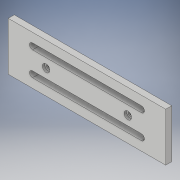
# Autodesk Inventor part: ps bottom
Saved by Autodesk Inventor 2017 (Build 210142000, 142)
## iProperties
Created: 2016-07-21
Part Number: ps bottom
Material: Generic
Document SubType Name: Modeling
Designer: Darien Morrow
Density: 1 g/cm^3
Appearance: Default
Author: Darien Morrow
Autodesk Inventor part; units mm, degrees
ref_plane "YZ Plane" through (0, 0, 0) normal (1, 0, 0) x (0, 1, 0)
ref_plane "XZ Plane" through (0, 0, 0) normal (0, 1, 0) x (-1, 0, 0)
ref_plane "XY Plane" through (0, 0, 0) normal (0, 0, 1) x (1, 0, 0)
sketch "Sketch1" plane through (0, 0, 0) normal (0, 0, 1) x (1, 0, 0)
  line L0 (0, 0) -> (165.1, 0)
  line L1 (165.1, 0) -> (165.1, 50.8)
  line L2 (165.1, 50.8) -> (0, 50.8)
  line L3 (0, 50.8) -> (0, 0)
  dimension "d0" = 165.1
  dimension "d1" = 50.8
  constraints: 8 end point, 2 parallel, 1 horizontal, 1 perpendicular
  measures "d0" distance between parallel lines of L1 L3
  measures "d1" distance between parallel lines of L0 L2
extrude "Extrusion1" add sketch "Sketch1" along normal blind 6.35
sketch "Sketch3" plane through (0, 0, 6.35) normal (0, 0, 1) x (1, 0, 0)
  line L0 (39.6875, 25.4) -> (125.4125, 25.4)
  line L1 (0, 0) -> (165.1, 0) projected
  line L2 (0, 50.8) -> (0, 0) projected
  line L3 (165.1, 50.8) -> (0, 50.8) projected
  line L4 (82.55, 50.8) -> (82.55, 0)
  line L5 (165.1, 0) -> (165.1, 50.8) projected
  dimension "d14" = 85.725
  dimension "d15" = 25.4
  dimension "d16" = 39.6875
  dimension "d33" = 165.1
  dimension "d34" = 39.6875
  constraints: 4 end point, 2 coincident, 2 midpoint, 1 horizontal
  measures "d14" distance of L0.end L0.start
  measures "d15" distance between parallel lines of L0 L1
  measures "d16" distance from line of L0.start L2
  measures "d33" distance of L1.start L1.end
  measures "d34" distance from line of L5 L0.end
hole "Hole1" at (39.6875, 25.4, 6.35) at (125.4125, 25.4, 6.35) direction (0, 0, -1) diameter 4.1656 depth 6.35 tip angle 118 counterbore diameter 7.9502 counterbore depth 2.54
sketch "Sketch4" plane through (0, 0, 0) normal (0, 0, -1) x (-1, 0, 0)
  line L0 (-139.7, 12.7) -> (-25.4, 12.7) construction
  line L1 (-139.7, 9.525) -> (-25.4, 9.525)
  line L2 (-25.4, 15.875) -> (-139.7, 15.875)
  arc A0 (-139.7, 15.875) -> (-139.7, 9.525) centre (-139.7, 12.7) ccw
  arc A1 (-25.4, 9.525) -> (-25.4, 15.875) centre (-25.4, 12.7) ccw
  line L3 (0, 50.8) -> (0, 0) projected
  line L4 (-139.7, 38.1) -> (-25.4, 38.1) construction
  line L5 (-139.7, 34.925) -> (-25.4, 34.925)
  line L6 (-25.4, 41.275) -> (-139.7, 41.275)
  arc A2 (-139.7, 41.275) -> (-139.7, 34.925) centre (-139.7, 38.1) ccw
  arc A3 (-25.4, 34.925) -> (-25.4, 41.275) centre (-25.4, 38.1) ccw
  line L7 (-165.1, 50.8) -> (0, 50.8) projected
  point P0 (-82.55, 12.7)
  point P1 (-82.55, 38.1)
  dimension "d24" = 6.35
  dimension "d25" = 25.4
  dimension "d26" = 114.3
  dimension "d27" = 6.35
  dimension "d28" = 25.4
  dimension "d29" = 12.7
  dimension "d32" = 114.3
  constraints: 16 end point, 8 point on circle, 8 tangent, 4 centre point, 2 horizontal, 2 midpoint, 2 parallel
  measures "d24" distance between parallel lines of L1 L2
  measures "d25" distance from line of L3 L0.end
  measures "d26" distance of L0.end L0.start
  measures "d27" diameter of A3
  measures "d28" distance of L0.end L4.end
  measures "d29" distance from line of L4.end L7
  measures "d32" distance of L4.end L4.start
extrude "Extrusion3" cut sketch "Sketch4" against normal blind 6.35
sketch "Sketch5" plane through (0, 0, 0) normal (0, 0, -1) x (-1, 0, 0)
  circle A0 centre (-39.6875, 25.4) radius 2.0828 projected
  circle A1 centre (-125.4125, 25.4) radius 2.0828 projected
  point P0 (0, 0)
  constraints: 2 coincident
hole "Hole2" at (39.6875, 25.4, 0) at (125.4125, 25.4, 0) direction (0, 0, 1) diameter 9.525 depth 2.54
body "Solid1"
